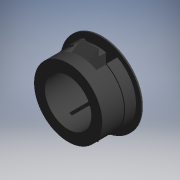
# Autodesk Inventor part: 8084904 CAFC-C6-T
Saved by Autodesk Inventor 2017.3 (Build 213256000, 256)
## iProperties
Part Number: 8084904 CAFC-C6-T
Material: Generic
Catalog Web Link: www.cadenas.de
Description: CAFC-C6 (c)-Protective cap
Vendor: FESTO
Document SubType Name: Modeling
Designer: partserver
Manufacturer: FESTO
Mass: 0.288896 g
Surface Area: 5.39766 cm^2
Volume: 0.288896 cm^3
Density: 1 g/cm^3
Appearance: PSOLRGB-80-80-80
Category: PARTsolutions
Company: FESTO
Title: 8084904 CAFC-C6-T
Author: Cadenas PARTsolutions
Comments: Protective cap
PSOL_IDENT_0: {$CADENAS_DATA\23d-libs\festo\parts\c\cafc\parts\cafc_c6_cap.prj},179 {VTYP=3D},{NB=8084904 CAFC-C6-
PSOL_IDENT_1: T},{LINA=8084904 CAFC-C6-T},{NN=CAFC-C6 (c)},{DATE=28.02.2020 13:07:36},{GEOMDATE=13.03.2018 12:29:0
PSOL_IDENT_2: 0},{VERSION=},{LINEID=10},{WBVAR=},{WBNUMERIC=}  {NB=8084904 CAFC-C6-T},{LINA=8084904 CAFC-C6-T},{KT=
PSOL_IDENT_3: DUMMY},{TNR=8084904},{TYP=CAFC-C6-T}
NB: 8084904 CAFC-C6-T
NN: CAFC-C6 (c)
NT: Protective cap
NBSYN: $TNR. $TYP.
LINA: 8084904 CAFC-C6-T
CATALOG: Festo
TNR: 8084904
TYP: CAFC-C6-T
SUPPLIER: FESTO
ARTICLENO: 8084904 CAFC-C6-T
BOMINFO: 8084904 CAFC-C6-T
CREATOR: CADENAS GmbH
Autodesk Inventor part; units mm, degrees
sketch "Sketch_1" plane through (0, 0, 0) normal (1, 0, 0) x (0, 1, 0)
  line L0 (0, 0) -> (6.4, 0)
  arc A0 (5, -5.95) -> (6.4, 0) centre (-9.5879, 0.6222) ccw
  line L1 (5, -5.95) -> (4.8, -5.95)
  line L2 (4.8, -5.95) -> (4.8, -5.15)
  line L3 (4.8, -5.15) -> (3.2, -5.15)
  line L4 (3.2, -5.15) -> (3.2, -5)
  line L5 (3.2, -5) -> (0, -5)
  line L6 (0, -5) -> (0, 0)
  line L7 (0, 0) -> (6.4, 0)
  constraints: 16 end point, 2 point on circle, 1 centre point
revolve "Revolution1" add sketch "Sketch_1" angle 360 about axis through (0, 0, 0) along (0, -1, 0)
sketch "Sketch_2" plane through (0, 0, 0) normal (1, 0, 0) x (0, 1, 0)
  line L0 (4.8, 0) -> (1.8, 0)
  line L1 (1.8, 0) -> (1.8, 5.15)
  line L2 (1.8, 5.15) -> (4.8, 5.15)
  line L3 (4.8, 5.15) -> (4.8, 0)
  line L4 (4.8, 0) -> (1.8, 0)
  constraints: 10 end point
revolve "Revolution2" cut sketch "Sketch_2" angle 57 mid plane about axis through (0, 4.8, 0) along (0, -1, 0)
sketch "Sketch_3" plane through (0, 0, 0) normal (1, 0, 0) x (0, 1, 0)
  line L0 (1.8, -0.1) -> (4.8, -0.1)
  line L1 (4.8, -0.1) -> (4.8, -5.25)
  line L2 (4.8, -5.25) -> (1.8, -5.25)
  line L3 (1.8, -5.25) -> (1.8, -0.1)
  line L4 (1.8, -0.1) -> (4.8, -0.1)
  constraints: 10 end point
revolve "Revolution3" cut sketch "Sketch_3" angle 57 mid plane about axis through (0, 1.8, -0.1) along (0, 1, 0)
sketch "Sketch_5" plane through (0, 0, 0) normal (1, 0, 0) x (0, 1, 0)
  line L0 (3.2, 5.95) -> (3.1, 5.95)
  line L1 (3.1, 5.95) -> (1.8, 4.8592)
  line L2 (1.8, 4.8592) -> (1.8, -4.8592)
  line L3 (1.8, -4.8592) -> (3.1, -5.95)
  line L4 (3.1, -5.95) -> (3.2, -5.95)
  line L5 (3.2, -5.95) -> (3.2, -5)
  line L6 (3.2, -5) -> (4.3, -5)
  line L7 (4.3, -5) -> (4.3, 5)
  line L8 (4.3, 5) -> (3.2, 5)
  line L9 (3.2, 5) -> (3.2, 5.95)
  constraints: 20 end point
extrude "Extrusion1" add sketch "Sketch_5" along normal mid plane 2.5
sketch "Sketch_6" plane through (0, 0, 0) normal (1, 0, 0) x (0, 1, 0)
  line L0 (4.5, 0) -> (4.3, 0)
  line L1 (4.3, 0) -> (4.3, 5)
  line L2 (4.3, 5) -> (3.2, 5)
  line L3 (3.2, 5) -> (3.2, 5.5)
  line L4 (3.2, 5.5) -> (4.5, 5.5)
  line L5 (4.5, 5.5) -> (4.5, 0)
  line L6 (4.5, 0) -> (4.3, 0)
  constraints: 14 end point
revolve "Revolution4" cut sketch "Sketch_6" angle 30 mid plane about axis through (0, 4.5, 0) along (0, -1, 0)
sketch "Sketch_7" plane through (0, 0, 0) normal (1, 0, 0) x (0, 1, 0)
  line L0 (4.3, 0) -> (4.5, 0)
  line L1 (4.3, -3) -> (4.3, -5)
  line L2 (4.3, -5) -> (3.2, -5)
  line L3 (3.2, -5) -> (3.2, -5.5)
  line L4 (3.2, -5.5) -> (4.5, -5.5)
  line L5 (4.5, -5.5) -> (4.5, -3)
  line L6 (4.5, -3) -> (4.3, -3)
  constraints: 14 end point
revolve "Revolution5" cut sketch "Sketch_7" angle 30 mid plane about axis through (0, 4.3, 0) along (0, 1, 0)
sketch "Sketch7" plane through (0, 0, 0) normal (0, -1, 0) x (1, 0, 0)
  point P0 (0, 0)
hole "Hole1" at (0, 0, 0) direction (0, 1, 0) diameter 6.8 depth 4.8
ref_plane "ANBAU_XY" through (0, 0, 0) normal (0, 1, 0) x (1, 0, 0)
ref_plane "ANBAU_YZ" through (0, 0, 0) normal (1, 0, 0) x (0, 0, -1)
ref_plane "ANBAU_ZX" through (0, 0, 0) normal (0, 0, -1) x (0, 1, 0)
body "Solid1"
